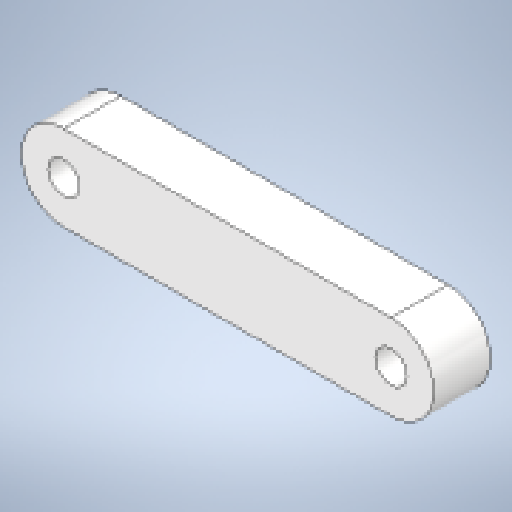
# Autodesk Inventor part: Sliders
Saved by Autodesk Inventor 2023.2 (Build 272271000, 271)
## iProperties
Created: 2024-01-14
Part Number: Sliders
Material: UHMW, White
Document SubType Name: Modeling
Designer: Nathan Cai
Density: 0.94 g/cm^3
Appearance: Smooth - White
Mass: 2.83732 g
Surface Area: 18.4507 cm^2
Volume: 3.01842 cm^3
Author: Nathan Cai
Autodesk Inventor part; units mm, degrees
ref_plane "YZ Plane" through (0, 0, 0) normal (1, 0, 0) x (0, 1, 0)
ref_plane "XZ Plane" through (0, 0, 0) normal (0, 1, 0) x (-1, 0, 0)
ref_plane "XY Plane" through (0, 0, 0) normal (0, 0, 1) x (1, 0, 0)
sketch "Sketch1" plane through (0, 0, 0) normal (0, 0, 1) x (1, 0, 0)
  line L0 (0, 0) -> (36.5125, 0) construction
  line L1 (0, -4.7625) -> (36.5125, -4.7625)
  line L2 (36.5125, 4.7625) -> (0, 4.7625)
  arc A0 (0, 4.7625) -> (0, -4.7625) centre (0, 0) ccw
  arc A1 (36.5125, -4.7625) -> (36.5125, 4.7625) centre (36.5125, 0) ccw
  circle A2 centre (0, 0) radius 1.7526
  circle A3 centre (36.5125, 0) radius 1.7526
  point P0 (18.2563, 0)
  dimension "d0" = 36.5125
  dimension "d1" = 9.525
  dimension "d2" = 3.5052
  dimension "d3" = 3.5052
  constraints: 8 end point, 4 centre point, 4 point on circle, 4 tangent, 2 coincident, 1 horizontal, 1 midpoint, 1 parallel
  measures "d0" distance of L0.start L0.end
  measures "d1" diameter of A1
  measures "d2" diameter of A2
  measures "d3" diameter of A3
extrude "Extrusion1" add sketch "Sketch1" along normal blind 6.35
equation "\"d0\" = Rail_Offset"
equation "\"d3\" = d2"
equation "\"Rail_Offset\" = 36.5125"
body "Solid1"
